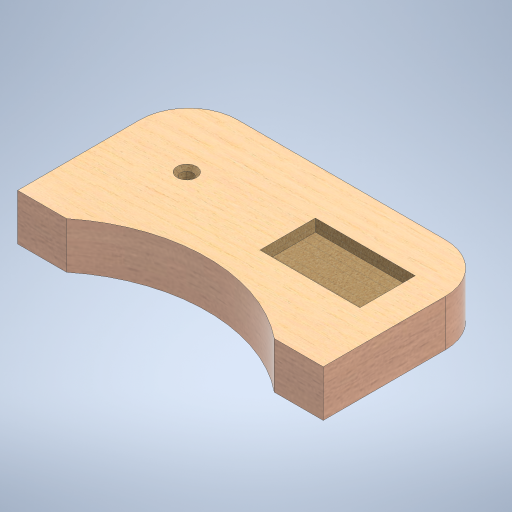
# Autodesk Inventor part: Demo Covering Queue 2
Saved by Autodesk Inventor 2024 (Build 280153000, 153)
## iProperties
Created: 2021-05-07
Part Number: Demo Covering Queue 2
Material: MLBRD
Document SubType Name: Modeling
Designer: sauliusd
Density: 0.8 g/cm^3
Appearance: MLMDF
Mass: 905.075 g
Surface Area: 940.533 cm^2
Volume: 1131.34 cm^3
Length: 250.0
Width: 140.0
Thickness: 38.0
Material Code: 2MDF
Front Edge: B01
Item Type: Part
Item_length: 250.0
Item_width: 140.0
Item_thickness: 38.0
Author: sauliusd
Autodesk Inventor part; units mm, degrees
ref_plane "YZ Plane" through (0, 0, 0) normal (1, 0, 0) x (0, 1, 0)
ref_plane "XZ Plane" through (0, 0, 0) normal (0, 1, 0) x (-1, 0, 0)
ref_plane "XY Plane" through (0, 0, 0) normal (0, 0, 1) x (1, 0, 0)
sketch "Sketch1" plane through (0, 0, 0) normal (0, 0, 1) x (1, 0, 0)
  line L0 (-125, -70) -> (125, -70)
  line L1 (125, -70) -> (125, 70)
  line L2 (125, 70) -> (-125, 70)
  line L3 (-125, 70) -> (-125, -70)
  line L4 (-125, -70) -> (125, 70) construction
  line L5 (125, -70) -> (-125, 70) construction
  point P0 (0, 0)
  dimension "d0" = 250
  dimension "d1" = 140
  constraints: 12 end point, 2 midpoint, 2 parallel, 1 horizontal, 1 perpendicular
  measures "d0" distance of L2.end L1.end
  measures "d1" distance of L1.end L0.end
extrude "Extrusion1" add sketch "Sketch1" along normal blind 38
sketch "Sketch2" plane through (0, 0, 38) normal (0, 0, 1) x (1, 0, 0)
  line L0 (125, -70) -> (125, 70) projected
  line L1 (125, 70) -> (-125, 70) projected
  line L2 (-125, 70) -> (-125, -70) projected
  line L3 (-125, -70) -> (125, -70) projected
  line L4 (-125, -70) -> (125, -70) projected
  arc A0 (85, -70) -> (-85, -70) centre (0, -175.4167) ccw
  line L5 (53.4733, -40) -> (-37.6413, -40) construction
  point P0 (0, 0)
  point P1 (85, -70)
  dimension "d5" = 40
  dimension "d114" = 30
  constraints: 2 end point, 2 point on circle, 2 point on line, 1 centre point, 1 horizontal, 1 tangent, 1 vertical alignment
  measures "d5" distance from line of L2 A0.end
  measures "d114" distance between parallel lines of L3 L5
extrude "Extrusion2" cut sketch "Sketch2" against normal through all contours L3 A0
fillet "Fillet1" radius 40 2 edges at (125, 70, 19) (-125, 70, 19)
sketch "Sketch3" plane through (0, 0, 38) normal (0, 0, 1) x (1, 0, 0)
  point P0 (0, 0)
  point P1 (-68.7955, 12.1981)
hole "Hole1" at (-68.7955, 12.1981, 38) direction (0, 0, -1) diameter 10 end through all countersink diameter 16 countersink angle 90
sketch "Sketch4" plane through (0, 0, 38) normal (0, 0, 1) x (1, 0, 0)
  line L0 (16.3939, 32.185) -> (98.1222, 32.185)
  line L1 (98.1222, 32.185) -> (98.1222, -13.1392)
  line L2 (98.1222, -13.1392) -> (16.3939, -13.1392)
  line L3 (16.3939, -13.1392) -> (16.3939, 32.185)
  point P0 (0, 0)
  constraints: 8 end point, 2 parallel, 1 horizontal, 1 perpendicular
extrude "Extrusion3" cut sketch "Sketch4" against normal blind 10
body "Solid1"
